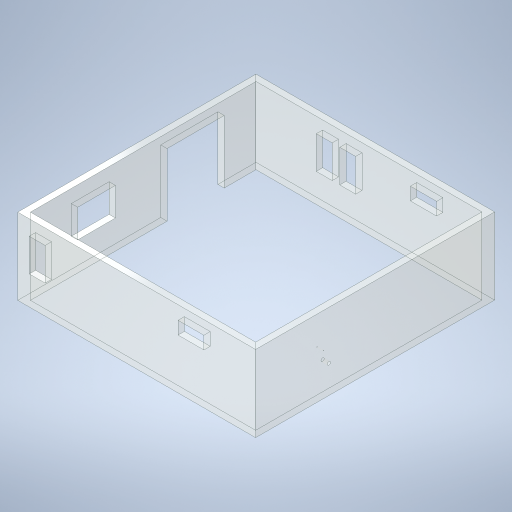
# Autodesk Inventor part: Exterior_Walls
Saved by Autodesk Inventor 2024 (Build 280153020, 153B)
## iProperties
Created: 2023-05-16
Part Number: Exterior_Walls
Material: Concrete
Document SubType Name: Modeling
Designer: Tom
Density: 2.40731 g/cm^3
Appearance: Clear
Mass: 3.19414e+07 g
Surface Area: 1.46557e+06 cm^2
Volume: 1.32685e+07 cm^3
Author: Tom
Autodesk Inventor part; units mm, degrees
ref_plane "YZ Plane" through (0, 0, 0) normal (1, 0, 0) x (0, 1, 0)
ref_plane "XZ Plane" through (0, 0, 0) normal (0, 1, 0) x (-1, 0, 0)
ref_plane "XY Plane" through (0, 0, 0) normal (0, 0, 1) x (1, 0, 0)
sketch "Sketch1" plane through (0, 0, 0) normal (0, 1, 0) x (-1, 0, 0)
  line L0 (0, 0) -> (12.7, 7213.5888)
  line L1 (12.7, 7213.5888) -> (7200.9, 7213.5888)
  line L2 (7200.9, 7213.5888) -> (7213.6, 0)
  line L3 (7213.6, 0) -> (0, 0)
  line L4 (7403.7426, 7416.7888) -> (-190.1426, 7416.7888)
  line L5 (-190.1426, 7416.7888) -> (-203.5581, -203.2)
  line L6 (-203.5581, -203.2) -> (7417.1581, -203.2)
  line L7 (7417.1581, -203.2) -> (7403.7426, 7416.7888)
  dimension "d1" = 7188.2
  dimension "d3" = 12.7
  dimension "d4" = 7213.6
  dimension "d5" = 7213.6
  dimension "d6" = 203.2
  dimension "d8" = 7213.6
  constraints: 16 end point, 1 horizontal, 3 other
  measures "d1" distance of L0.end L1.end
  measures "d3" horizontal distance of L0.start L0.end
  measures "d4" distance of L1.end L2.end
  measures "d5" distance of L2.end L0.start
  measures "d6" distance between parallel lines of L4 L1
  measures "d8" distance of L0.start L0.end
extrude "Extrusion1" add sketch "Sketch1" along normal blind 2438.4
sketch "Sketch4" plane through (-12.7, 0, 7213.5888) normal (-0.9999985, 0, -0.0017606) x (-0.0017606, 0, 0.9999985)
  line L0 (-7213.6, 0) -> (0, 0) projected
  line L1 (-7213.6, 0) -> (-7213.6, 2438.4) projected
  point P0 (-1955.8, 1330.325)
  dimension "d27" = 1330.325
  dimension "d28" = 5257.8
  measures "d27" distance from line of L0 point (-1955.8, 1330.325)
  measures "d28" distance from line of L1 point (-1955.8, 1330.325)
hole "Hole1" at (-9.2567, 1330.325, 5257.7919) direction (0.9999985, 0, 0.0017606) diameter 19.05 end through all
sketch "Sketch5" plane through (-12.7, 0, 7213.5888) normal (-0.9999985, 0, -0.0017606) x (-0.0017606, 0, 0.9999985)
  line L0 (-7213.6, 0) -> (0, 0) projected
  line L1 (-7213.6, 0) -> (-7213.6, 2438.4) projected
  point P0 (-2133.6, 889)
  dimension "d36" = 889
  dimension "d37" = 5080
  measures "d36" distance from line of L0 point (-2133.6, 889)
  measures "d37" distance from line of L1 point (-2133.6, 889)
hole "Hole2" at (-8.9437, 889, 5079.9921) direction (0.9999985, 0, 0.0017606) diameter 101.6 end through all
sketch "Sketch6" plane through (-7213.6, 0, 0) normal (0, 0, 1) x (1, 0, 0)
  line L0 (7417.1581, 2438.4) -> (-203.5581, 2438.4) projected
  line L1 (7213.6, 0) -> (7213.6, 2438.4) projected
  line L2 (0, 0) -> (7213.6, 0) projected
  line L3 (4927.6, 2006.6) -> (5765.8, 2006.6)
  line L4 (5765.8, 2006.6) -> (5765.8, 1600.2)
  line L5 (5765.8, 1600.2) -> (4927.6, 1600.2)
  line L6 (4927.6, 1600.2) -> (4927.6, 2006.6)
  dimension "d119" = 1447.8
  dimension "d121" = 406.4
  dimension "d136" = 838.2
  dimension "d137" = 1600.2
  constraints: 8 end point, 2 parallel, 1 horizontal, 1 perpendicular
  measures "d119" distance between parallel lines of L1 L4
  measures "d121" distance of L5.end L3.start
  measures "d136" distance of L3.start L3.end
  measures "d137" distance between parallel lines of L2 L5
extrude "Extrusion3" cut sketch "Sketch6" against normal up to surface (203.2 mm away)
sketch "Sketch7" plane through (-7213.6, 0, 0) normal (0.9999985, 0, -0.0017606) x (-0.0017606, 0, -0.9999985)
  line L0 (-7213.6, 0) -> (0, 0) projected
  line L1 (-1016, 0) -> (-2844.8, 0)
  line L2 (-2844.8, 0) -> (-2844.8, 2006.6)
  line L3 (-2844.8, 2006.6) -> (-1016, 2006.6)
  line L4 (-1016, 2006.6) -> (-1016, 0)
  line L5 (0, 0) -> (0, 2438.4) projected
  point P0 (-12.7, 0)
  point P1 (-2844.8, 0)
  dimension "d51" = 1016
  dimension "d52" = 2006.6
  dimension "d53" = 1828.8
  constraints: 8 end point, 2 parallel, 1 horizontal, 1 perpendicular, 1 point on line
  measures "d51" distance between parallel lines of L5 L4
  measures "d52" distance of L1.end L2.end
  measures "d53" distance of L2.end L3.end
extrude "Extrusion4" cut sketch "Sketch7" against normal up to surface (203.2 mm away)
sketch "Sketch8" plane through (-7200.9, 0, 7213.5888) normal (0.9999985, 0, -0.0017606) x (-0.0017606, 0, -0.9999985)
  line L0 (2717.8, 1816.1) -> (1511.3, 1816.1)
  line L1 (1511.3, 1816.1) -> (1511.3, 914.4)
  line L2 (1511.3, 914.4) -> (2717.8, 914.4)
  line L3 (2717.8, 914.4) -> (2717.8, 1816.1)
  line L4 (0, 0) -> (0, 2438.4) projected
  line L5 (0, 0) -> (4368.8, 0) projected
  point P0 (7200.9, 0)
  dimension "d27" = 1330.325
  dimension "d56" = 2717.8
  dimension "d57" = 1206.5
  dimension "d58" = 901.7
  dimension "d59" = 914.4
  constraints: 8 end point, 2 parallel, 1 horizontal, 1 perpendicular
  measures "d56" distance between parallel lines of L4 L3
  measures "d57" distance of L1.end L2.end
  measures "d58" distance of L0.end L1.end
  measures "d59" distance between parallel lines of L5 L2
extrude "Extrusion5" cut sketch "Sketch8" against normal up to surface (203.2 mm away)
sketch "Sketch9" plane through (-7213.6, 0, 0) normal (0, 0, 1) x (1, 0, 0)
  line L0 (3181.5024, 1955.8) -> (2673.5024, 1955.8)
  line L1 (2673.5024, 1955.8) -> (2673.5024, 914.4)
  line L2 (2673.5024, 914.4) -> (3181.5024, 914.4)
  line L3 (3181.5024, 914.4) -> (3181.5024, 1955.8)
  line L4 (0, 0) -> (7213.6, 0) projected
  line L5 (7213.6, 0) -> (7213.6, 2438.4) projected
  dimension "d63" = 1041.4
  dimension "d64" = 508
  dimension "d65" = 914.4
  dimension "d66" = 4540.0976
  constraints: 8 end point, 2 parallel, 1 horizontal, 1 perpendicular
  measures "d63" distance of L2.end L0.start
  measures "d64" distance between parallel lines of L1 L3
  measures "d65" distance between parallel lines of L4 L2
  measures "d66" distance between parallel lines of L5 L1
extrude "Extrusion6" cut sketch "Sketch9" against normal up to surface (203.2 mm away)
sketch "Sketch10" plane through (-7213.6, 0, 0) normal (0, 0, 1) x (1, 0, 0)
  line L0 (2432.2024, 914.4) -> (1924.2024, 914.4)
  line L1 (1924.2024, 914.4) -> (1924.2024, 1955.8)
  line L2 (1924.2024, 1955.8) -> (2432.2024, 1955.8)
  line L3 (2432.2024, 1955.8) -> (2432.2024, 914.4)
  line L4 (0, 0) -> (7213.6, 0) projected
  line L5 (0, 0) -> (0, 2438.4) projected
  dimension "d69" = 914.4
  dimension "d70" = 1041.4
  dimension "d71" = 508
  dimension "d72" = 1924.2024
  constraints: 8 end point, 2 parallel, 1 horizontal, 1 perpendicular
  measures "d69" distance between parallel lines of L4 L0
  measures "d70" distance of L2.end L0.start
  measures "d71" distance of L0.start L0.end
  measures "d72" distance between parallel lines of L5 L1
extrude "Extrusion7" cut sketch "Sketch10" against normal up to surface (203.2 mm away)
sketch "Sketch11" plane through (-12.7, 0, 7213.5888) normal (0, 0, -1) x (-1, 0, 0)
  line L0 (7023.2524, 914.4) -> (6515.2524, 914.4)
  line L1 (6515.2524, 914.4) -> (6515.2524, 1955.8)
  line L2 (6515.2524, 1955.8) -> (7023.2524, 1955.8)
  line L3 (7023.2524, 1955.8) -> (7023.2524, 914.4)
  line L4 (7188.2, 0) -> (7188.2, 2438.4) projected
  line L5 (0, 0) -> (7188.2, 0) projected
  point P0 (-12.7, 0)
  dimension "d75" = 164.9476
  dimension "d76" = 1041.4
  dimension "d79" = 508
  dimension "d80" = 914.4
  constraints: 8 end point, 2 parallel, 1 horizontal, 1 perpendicular
  measures "d75" distance between parallel lines of L4 L3
  measures "d76" distance of L0.end L1.end
  measures "d79" distance between parallel lines of L3 L1
  measures "d80" distance between parallel lines of L5 L0
extrude "Extrusion8" cut sketch "Sketch11" against normal up to surface (203.2 mm away)
sketch "Sketch20" plane through (-7403.7426, 0, 7416.7888) normal (0, 0, 1) x (1, 0, 0)
  line L0 (5117.7426, 2006.6) -> (5943.2426, 2006.6)
  line L1 (5943.2426, 2006.6) -> (5943.2426, 1600.2)
  line L2 (5943.2426, 1600.2) -> (5117.7426, 1600.2)
  line L3 (5117.7426, 1600.2) -> (5117.7426, 2006.6)
  line L4 (0, 2438.4) -> (7593.8851, 2438.4) projected
  line L5 (0, 0) -> (7593.8851, 0) projected
  point P0 (7403.7426, 0)
  point P1 (7391.0426, 2438.4)
  dimension "d129" = 406.4
  dimension "d134" = 825.5
  dimension "d135" = 1600.2
  dimension "d138" = 1447.8
  constraints: 8 end point, 2 parallel, 1 horizontal, 1 perpendicular
  measures "d129" distance of L2.end L0.start
  measures "d134" distance of L0.start L0.end
  measures "d135" distance between parallel lines of L5 L2
  measures "d138" distance from line of L1 point (7391.043, 2438.4)
extrude "Extrusion16" cut sketch "Sketch20" against normal up to surface (203.2 mm away)
body "Solid1"
